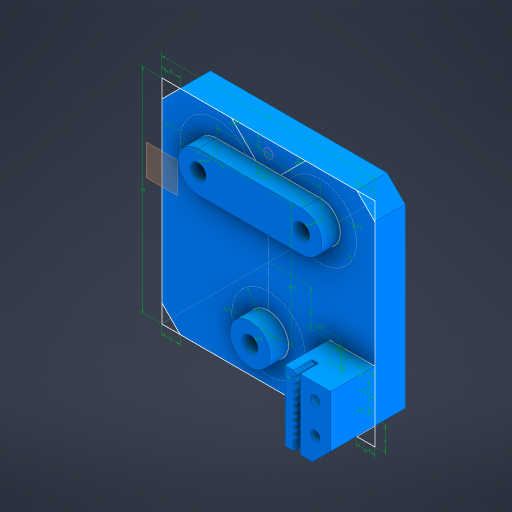
# Autodesk Inventor part: Toolhead
Saved by Autodesk Inventor 2024.2 (Build 282272000, 272)
## iProperties
Created: 2024-10-16
Part Number: Toolhead
Material: Generic
Document SubType Name: Modeling
Designer: jerem
Density: 1 g/cm^3
Appearance: Default
Author: jerem
## iProperties of the stored document Toolhead_3DPrint.ipt
Created: 2024-10-16
Part Number: Toolhead_3DPrint
Material: Generic
Document SubType Name: Modeling
Designer: jerem
Density: 1 g/cm^3
Appearance: Default
Author: jerem
Autodesk Inventor part; units mm, degrees
ref_plane "YZ Plane" through (0, 0, 0) normal (1, 0, 0) x (0, 1, 0)
ref_plane "XZ Plane" through (0, 0, 0) normal (0, 1, 0) x (-1, 0, 0)
ref_plane "XY Plane" through (0, 0, 0) normal (0, 0, 1) x (1, 0, 0)
sketch "Sketch1" plane through (0, 0, 0) normal (0, 0, 1) x (1, 0, 0)
  line L0 (0, 0) -> (0, 20.25) construction
  line L1 (0, 0) -> (0, -20.25) construction
  line L2 (0, 20.25) -> (-17, 20.25) construction
  line L3 (0, 20.25) -> (17, 20.25) construction
  circle A0 centre (-17, 20.25) radius 2.6
  circle A1 centre (17, 20.25) radius 2.6
  circle A2 centre (0, -20.25) radius 2.6
  circle A3 centre (-17, 20.25) radius 6.6
  circle A4 centre (17, 20.25) radius 6.6
  circle A5 centre (0, -20.25) radius 6.6
  circle A6 centre (-17, 20.25) radius 12 construction
  circle A7 centre (17, 20.25) radius 12 construction
  circle A8 centre (0, -20.25) radius 12 construction
  line L4 (35, -35) -> (-35, -35)
  line L5 (-35, -35) -> (-35, 35)
  line L6 (-35, 35) -> (35, 35)
  line L7 (35, 35) -> (35, -35)
  line L8 (-35, -35) -> (35, 35) construction
  line L9 (35, -35) -> (35, -35)
  line L10 (35, -35) -> (35, -12)
  line L11 (35, -12) -> (35, -12)
  line L12 (35, -12) -> (35, -35)
  line L13 (-17, 26.85) -> (17, 26.85)
  line L14 (-17, 13.65) -> (17, 13.65)
  line L15 (-35, 29) -> (-29, 35)
  line L16 (29, 35) -> (35, 29)
  line L17 (35, -29) -> (29, -35)
  line L18 (-29, -35) -> (-35, -29)
  arc A9 (22.85, -12) -> (23.3073, -12.5421) centre (23.4, -12) ccw
  line L19 (23.4, -12) -> (22.85, -12) construction
  line L20 (22.85, -12) -> (20, -12)
  line L21 (23.3073, -12.5421) -> (23.7921, -12.625)
  arc A10 (24, -12.8714) -> (23.7921, -12.625) centre (23.75, -12.8714) ccw
  line L22 (24, -13) -> (23.4, -13) construction
  line L23 (24, -13.1286) -> (24, -12.8714)
  arc A11 (23.7921, -13.375) -> (24, -13.1286) centre (23.75, -13.1286) ccw
  line L24 (23.7921, -13.375) -> (23.3073, -13.4579)
  line L25 (20, -12) -> (20, -14)
  line L26 (22.85, -14) -> (20, -14) construction
  line L27 (23.4, -14) -> (23.4, -12) construction
  arc A12 (23.3073, -13.4579) -> (22.85, -14) centre (23.4, -14) ccw
  line L28 (25, -12) -> (25, -35)
  line L29 (25, -12) -> (35, -12)
  line L30 (22.85, -14) -> (20, -14)
  arc A13 (22.85, -14) -> (23.3073, -14.5421) centre (23.4, -14) ccw
  line L31 (23.3073, -14.5421) -> (23.7921, -14.625)
  line L32 (20, -14) -> (20, -16)
  line L33 (22.85, -16) -> (20, -16) construction
  line L34 (24, -15) -> (23.4, -15) construction
  line L35 (24, -15.1286) -> (24, -14.8714)
  line L36 (23.7921, -15.375) -> (23.3073, -15.4579)
  arc A14 (23.3073, -15.4579) -> (22.85, -16) centre (23.4, -16) ccw
  arc A15 (23.7921, -15.375) -> (24, -15.1286) centre (23.75, -15.1286) ccw
  arc A16 (24, -14.8714) -> (23.7921, -14.625) centre (23.75, -14.8714) ccw
  line L37 (22.85, -16) -> (20, -16) construction
  arc A17 (22.85, -16) -> (23.3073, -16.5421) centre (23.4, -16) ccw
  line L38 (23.3073, -16.5421) -> (23.7921, -16.625)
  line L39 (20, -16) -> (20, -18)
  line L40 (22.85, -18) -> (20, -18) construction
  line L41 (24, -17) -> (23.4, -17) construction
  line L42 (24, -17.1286) -> (24, -16.8714)
  line L43 (23.7921, -17.375) -> (23.3073, -17.4579)
  arc A18 (23.3073, -17.4579) -> (22.85, -18) centre (23.4, -18) ccw
  arc A19 (23.7921, -17.375) -> (24, -17.1286) centre (23.75, -17.1286) ccw
  arc A20 (24, -16.8714) -> (23.7921, -16.625) centre (23.75, -16.8714) ccw
  line L44 (22.85, -18) -> (20, -18) construction
  arc A21 (22.85, -18) -> (23.3073, -18.5421) centre (23.4, -18) ccw
  line L45 (23.3073, -18.5421) -> (23.7921, -18.625)
  line L46 (20, -18) -> (20, -20)
  line L47 (22.85, -20) -> (20, -20) construction
  line L48 (24, -19) -> (23.4, -19) construction
  line L49 (24, -19.1286) -> (24, -18.8714)
  line L50 (23.7921, -19.375) -> (23.3073, -19.4579)
  arc A22 (23.3073, -19.4579) -> (22.85, -20) centre (23.4, -20) ccw
  arc A23 (23.7921, -19.375) -> (24, -19.1286) centre (23.75, -19.1286) ccw
  arc A24 (24, -18.8714) -> (23.7921, -18.625) centre (23.75, -18.8714) ccw
  line L51 (22.85, -20) -> (20, -20) construction
  arc A25 (22.85, -20) -> (23.3073, -20.5421) centre (23.4, -20) ccw
  line L52 (23.3073, -20.5421) -> (23.7921, -20.625)
  line L53 (20, -20) -> (20, -22)
  line L54 (22.85, -22) -> (20, -22) construction
  line L55 (24, -21) -> (23.4, -21) construction
  line L56 (24, -21.1286) -> (24, -20.8714)
  line L57 (23.7921, -21.375) -> (23.3073, -21.4579)
  arc A26 (23.3073, -21.4579) -> (22.85, -22) centre (23.4, -22) ccw
  arc A27 (23.7921, -21.375) -> (24, -21.1286) centre (23.75, -21.1286) ccw
  arc A28 (24, -20.8714) -> (23.7921, -20.625) centre (23.75, -20.8714) ccw
  line L58 (22.85, -22) -> (20, -22) construction
  arc A29 (22.85, -22) -> (23.3073, -22.5421) centre (23.4, -22) ccw
  line L59 (23.3073, -22.5421) -> (23.7921, -22.625)
  line L60 (20, -22) -> (20, -24)
  line L61 (22.85, -24) -> (20, -24) construction
  line L62 (24, -23) -> (23.4, -23) construction
  line L63 (24, -23.1286) -> (24, -22.8714)
  line L64 (23.7921, -23.375) -> (23.3073, -23.4579)
  arc A30 (23.3073, -23.4579) -> (22.85, -24) centre (23.4, -24) ccw
  arc A31 (23.7921, -23.375) -> (24, -23.1286) centre (23.75, -23.1286) ccw
  arc A32 (24, -22.8714) -> (23.7921, -22.625) centre (23.75, -22.8714) ccw
  line L65 (22.85, -24) -> (20, -24) construction
  arc A33 (22.85, -24) -> (23.3073, -24.5421) centre (23.4, -24) ccw
  line L66 (23.3073, -24.5421) -> (23.7921, -24.625)
  line L67 (20, -24) -> (20, -26)
  line L68 (22.85, -26) -> (20, -26) construction
  line L69 (24, -25) -> (23.4, -25) construction
  line L70 (24, -25.1286) -> (24, -24.8714)
  line L71 (23.7921, -25.375) -> (23.3073, -25.4579)
  arc A34 (23.3073, -25.4579) -> (22.85, -26) centre (23.4, -26) ccw
  arc A35 (23.7921, -25.375) -> (24, -25.1286) centre (23.75, -25.1286) ccw
  arc A36 (24, -24.8714) -> (23.7921, -24.625) centre (23.75, -24.8714) ccw
  line L72 (22.85, -26) -> (20, -26) construction
  arc A37 (22.85, -26) -> (23.3073, -26.5421) centre (23.4, -26) ccw
  line L73 (23.3073, -26.5421) -> (23.7921, -26.625)
  line L74 (20, -26) -> (20, -28)
  line L75 (22.85, -28) -> (20, -28) construction
  line L76 (24, -27) -> (23.4, -27) construction
  line L77 (24, -27.1286) -> (24, -26.8714)
  line L78 (23.7921, -27.375) -> (23.3073, -27.4579)
  arc A38 (23.3073, -27.4579) -> (22.85, -28) centre (23.4, -28) ccw
  arc A39 (23.7921, -27.375) -> (24, -27.1286) centre (23.75, -27.1286) ccw
  arc A40 (24, -26.8714) -> (23.7921, -26.625) centre (23.75, -26.8714) ccw
  line L79 (22.85, -28) -> (20, -28) construction
  arc A41 (22.85, -28) -> (23.3073, -28.5421) centre (23.4, -28) ccw
  line L80 (23.3073, -28.5421) -> (23.7921, -28.625)
  line L81 (20, -28) -> (20, -30)
  line L82 (22.85, -30) -> (20, -30) construction
  line L83 (24, -29) -> (23.4, -29) construction
  line L84 (24, -29.1286) -> (24, -28.8714)
  line L85 (23.7921, -29.375) -> (23.3073, -29.4579)
  arc A42 (23.3073, -29.4579) -> (22.85, -30) centre (23.4, -30) ccw
  arc A43 (23.7921, -29.375) -> (24, -29.1286) centre (23.75, -29.1286) ccw
  arc A44 (24, -28.8714) -> (23.7921, -28.625) centre (23.75, -28.8714) ccw
  line L86 (22.85, -30) -> (20, -30) construction
  arc A45 (22.85, -30) -> (23.3073, -30.5421) centre (23.4, -30) ccw
  line L87 (23.3073, -30.5421) -> (23.7921, -30.625)
  line L88 (20, -30) -> (20, -32)
  line L89 (22.85, -32) -> (20, -32) construction
  line L90 (24, -31) -> (23.4, -31) construction
  line L91 (24, -31.1286) -> (24, -30.8714)
  line L92 (23.7921, -31.375) -> (23.3073, -31.4579)
  arc A46 (23.3073, -31.4579) -> (22.85, -32) centre (23.4, -32) ccw
  arc A47 (23.7921, -31.375) -> (24, -31.1286) centre (23.75, -31.1286) ccw
  arc A48 (24, -30.8714) -> (23.7921, -30.625) centre (23.75, -30.8714) ccw
  circle A49 centre (30, -27) radius 1.5
  line L93 (22.85, -12) -> (25, -12)
  circle A50 centre (30, -17) radius 1.5
  line L94 (30, -17) -> (30, -27) construction
  line L95 (20, -32) -> (20, -35)
  line L96 (22.85, -32) -> (22.85, -35)
  line L97 (-12.15, 35) -> (-4, 26.85)
  line L98 (4, 26.85) -> (12.15, 35)
  circle A51 centre (0, 31) radius 1.5
  point P0 (30, -4)
  point P1 (35, -12)
  point P2 (22.85, -30)
  point P3 (22.85, -28)
  point P4 (22.85, -26)
  point P5 (22.85, -24)
  point P6 (22.85, -22)
  point P7 (22.85, -20)
  point P8 (22.85, -18)
  point P9 (22.85, -16)
  point P10 (0, 26.85)
  dimension "d19" = 5.2
  dimension "d20" = 5.2
  dimension "d21" = 5.2
  dimension "d22" = 4
  dimension "d23" = 4
  dimension "d24" = 4
  dimension "d25" = 40.5
  dimension "d26" = 34
  dimension "d27" = 24
  dimension "d28" = 24
  dimension "d29" = 24
  dimension "d43" = 70
  dimension "d44" = 70
  dimension "d123" = 6
  dimension "d124" = 6
  dimension "d125" = 6
  dimension "d126" = 6
  dimension "d136" = 1.1
  dimension "d137" = 2
  dimension "d138" = 0.25
  dimension "d139" = -0.75
  dimension "d140" = 1.15
  dimension "d141" = 1
  dimension "d142" = 2
  dimension "d143" = 3
  dimension "d144" = 3
  dimension "d145" = 5
  dimension "d146" = 10
  dimension "d149" = 5
  dimension "d150" = 10
  dimension "d151" = 8
  dimension "d158" = 12
  dimension "d160" = 45
  dimension "d161" = 45
  dimension "d162" = 8
  dimension "d164" = 4
  dimension "d165" = 3
  dimension "d166" = 4
  dimension "d37" = 1.1
  dimension "d38" = 1.1
  dimension "d39" = 2
  dimension "d40" = 0.25
  dimension "d41" = -0.75
  dimension "d50" = 12
  dimension "d51" = 1.15
  dimension "d57" = 1
  dimension "d65" = 2
  dimension "d71" = 3
  dimension "d89" = 3
  dimension "d92" = 5
  dimension "d107" = 25
  dimension "d108" = 45
  dimension "d109" = 45
  dimension "d110" = 10
  dimension "d111" = 10
  dimension "d112" = 7
  dimension "d119" = 3
  dimension "d120" = 3
  dimension "d121" = 3
  dimension "d127" = 5
  dimension "d128" = 10
  dimension "d129" = 8
  dimension "d130" = 10
  constraints: 198 end point, 85 point on circle, 52 centre point, 17 point on line, 12 perpendicular, 9 coincident, 8 horizontal, 8 tangent, 6 vertical, 4 collinear, 4 midpoint, 4 parallel, 2 line through centre, 1 equal radius, 243 other
  measures "d19" diameter of A0
  measures "d20" diameter of A1
  measures "d21" diameter of A2
  measures "d22" radial gap between concentric circles of A3 A0
  measures "d23" radial gap between concentric circles of A4 A1
  measures "d24" radial gap between concentric circles of A5 A2
  measures "d25" distance of L1.end L0.end
  measures "d26" distance of L3.end L2.end
  measures "d27" diameter of A6
  measures "d28" diameter of A7
  measures "d29" diameter of A8
  measures "d43" distance of L5.end L6.end
  measures "d44" distance of L4.end L5.end
  measures "d123" distance of L4.end L18.start
  measures "d124" distance of L9.end L17.end
  measures "d125" distance of L16.start L6.end
  measures "d126" distance of L5.end L15.end
  measures "d136" diameter of A9
  measures "d137" distance of L27.end L27.start
  measures "d138" radius of A11
  measures "d139" distance of L21.end L24.start
  measures "d140" horizontal distance of L93.start L22.start
  measures "d141" distance between parallel lines of L28 L23
  measures "d142" distance of L27.end A13.centre
  measures "d143" diameter of A49
  measures "d144" diameter of A50
  measures "d145" distance between parallel lines of L28 L25
  measures "d146" distance of L94.start L94.end
  measures "d149" distance between parallel lines of L7 L94
  measures "d150" distance between parallel lines of L7 L28
  measures "d151" distance from line of L4 L94.end
  measures "d158" vertical distance of L20.end L0.start
  measures "d160" angle of L6 L97
  measures "d161" angle of L6 L98
  measures "d162" distance of L98.start L97.end
  measures "d164" distance of L97.end point (0, 26.85)
  measures "d165" diameter of A51
  measures "d166" distance from line of L6 A51.centre
extrude "Extrusion1" add sketch "Sketch1" against normal blind 10 contours A3 | A3 L13 A4 L14 | A3 L14 A4 L13 L98 L6 L16 L7 L29 L93 L20 L25 L32 L39 L46 L53 L60 L67 L74 L81 L88 L95 L4 L18 L5 L15 L97 | L97 L6 L98 L13 | A4 | L7 L17 L4 L28 L29 | L28 L4 L96 A46 L92 A47 L91 A48 L87 A45 A42 L85 A43 L84 A44 L80 A41 A38 L78 A39 L77 A40 L73 A37 A34 L71 A35 L70 A36 L66 A33 A30 L64 A31 L63 A32 L59 A29 A26 L57 A27 L56 A28 L52 A25 A22 L50 A23 L49 A24 L45 A21 A18 L43 A19 L42 A20 L38 A17 A14 L36 A15 L35 A16 L31 A13 A12 L24 A11 L23 A10 L21 A9 L93 | L95 L88 L81 L74 L67 L60 L53 L46 L39 L32 L30 A13 L31 A16 L35 A15 L36 A14 A17 L38 A20 L42 A19 L43 A18 A21 L45 A24 L49 A23 L50 A22 A25 L52 A28 L56 A27 L57 A26 A29 L59 A32 L63 A31 L64 A30 A33 L66 A36 L70 A35 L71 A34 A37 L73 A40 L77 A39 L78 A38 A41 L80 A44 L84 A43 L85 A42 A45 L87 A48 L91 A47 L92 A46 L96 L4 | A9 L21 A10 L23 A11 L24 A12 L30 L25 L20 | A5 | A51
extrude "Extrusion2" add sketch "Sketch1" along normal blind 6 contours A3 | A4 | A5
ref_plane "Work Plane1" through (17, 20.25, 11.5) normal (0, 0, 1) x (1, 0, 0)
extrude "Extrusion9" add sketch "Sketch1" along normal mid plane 6 from surface at 11.5 contours L7 L17 L4 L28 L29 | L95 L88 L81 L74 L67 L60 L53 L46 L39 L32 L30 A13 L31 A16 L35 A15 L36 A14 A17 L38 A20 L42 A19 L43 A18 A21 L45 A24 L49 A23 L50 A22 A25 L52 A28 L56 A27 L57 A26 A29 L59 A32 L63 A31 L64 A30 A33 L66 A36 L70 A35 L71 A34 A37 L73 A40 L77 A39 L78 A38 A41 L80 A44 L84 A43 L85 A42 A45 L87 A48 L91 A47 L92 A46 L96 L4 | A9 L21 A10 L23 A11 L24 A12 L30 L25 L20
extrude "Extrusion10" add sketch "Sketch1" along normal up to surface (8.5 mm away) contours L7 L17 L4 L28 L29 | L28 L4 L96 A46 L92 A47 L91 A48 L87 A45 A42 L85 A43 L84 A44 L80 A41 A38 L78 A39 L77 A40 L73 A37 A34 L71 A35 L70 A36 L66 A33 A30 L64 A31 L63 A32 L59 A29 A26 L57 A27 L56 A28 L52 A25 A22 L50 A23 L49 A24 L45 A21 A18 L43 A19 L42 A20 L38 A17 A14 L36 A15 L35 A16 L31 A13 A12 L24 A11 L23 A10 L21 A9 L93 | L95 L88 L81 L74 L67 L60 L53 L46 L39 L32 L30 A13 L31 A16 L35 A15 L36 A14 A17 L38 A20 L42 A19 L43 A18 A21 L45 A24 L49 A23 L50 A22 A25 L52 A28 L56 A27 L57 A26 A29 L59 A32 L63 A31 L64 A30 A33 L66 A36 L70 A35 L71 A34 A37 L73 A40 L77 A39 L78 A38 A41 L80 A44 L84 A43 L85 A42 A45 L87 A48 L91 A47 L92 A46 L96 L4 | A9 L21 A10 L23 A11 L24 A12 L30 L25 L20
extrude "Extrusion11" add sketch "Sketch1" along normal blind 6 contours A3 L13 A4 L14
sketch "Sketch3" plane through (0, 0, -10) normal (0, 0, -1) x (-1, 0, 0)
  circle A0 centre (0, -20.25) radius 2.6 construction
  circle A1 centre (0, -20.25) radius 5 construction
  circle A2 centre (0, -20.25) radius 6.6 projected
  line L0 (-2.5, -15.9199) -> (2.5, -15.9199)
  line L1 (2.5, -15.9199) -> (5, -20.25)
  line L2 (5, -20.25) -> (2.5, -24.5801)
  line L3 (2.5, -24.5801) -> (-2.5, -24.5801)
  line L4 (-2.5, -24.5801) -> (-5, -20.25)
  line L5 (-5, -20.25) -> (-2.5, -15.9199)
  dimension "d94" = 10
  constraints: 12 end point, 2 coincident, 1 horizontal, 16 other
equation "\"d20\" = d19"
equation "\"d21\" = d19"
equation "\"d23\" = d22"
equation "\"d24\" = d22"
body "Solid1"
